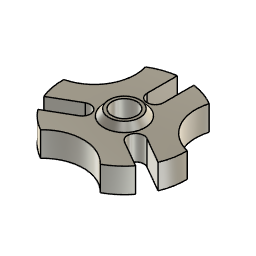
exercise13 (Autodesk Fusion 360 design; units mm, degrees)
Autodesk Fusion 360 part; units mm, degrees
sketch "草图1" plane through (0, 0, 0) normal (0, 0, 1) x (1, 0, 0)
  line L0 (0, 100) -> (0, -123.0461) construction
  line L1 (-180, 0) -> (103.1908, 0) construction
  arc A0 (14.5237, -26.25) -> (-14.5237, -26.25) centre (0, -40) ccw
  line L2 (-4, 29.7321) -> (-4, 15)
  line L3 (4, 15) -> (4, 29.7321)
  arc A1 (-4, 15) -> (0, 11) centre (0, 15) ccw
  arc A2 (0, 11) -> (4, 15) centre (0, 15) ccw
  line L4 (-14.9904, -4.0359) -> (-27.7488, -11.402)
  line L5 (-23.7488, -18.3302) -> (-10.9904, -10.9641)
  arc A3 (-10.9904, -10.9641) -> (-9.5263, -5.5) centre (-12.9904, -7.5) ccw
  arc A4 (-9.5263, -5.5) -> (-14.9904, -4.0359) centre (-12.9904, -7.5) ccw
  arc A5 (15.4713, 25.7029) -> (29.995, 0.5471) centre (34.641, 20) ccw
  line L6 (10.9904, -10.9641) -> (23.7488, -18.3302)
  line L7 (27.7488, -11.402) -> (14.9904, -4.0359)
  arc A6 (14.9904, -4.0359) -> (9.5263, -5.5) centre (12.9904, -7.5) ccw
  arc A7 (9.5263, -5.5) -> (10.9904, -10.9641) centre (12.9904, -7.5) ccw
  arc A8 (-29.995, 0.5471) -> (-15.4713, 25.7029) centre (-34.641, 20) ccw
  arc A9 (15.4713, 25.7029) -> (4, 29.7321) centre (0, 0) ccw
  arc A10 (-4, 29.7321) -> (-15.4713, 25.7029) centre (0, 0) ccw
  arc A11 (27.7488, -11.402) -> (29.995, 0.5471) centre (0, 0) ccw
  arc A12 (14.5237, -26.25) -> (23.7488, -18.3302) centre (0, 0) ccw
  arc A13 (-29.995, 0.5471) -> (-27.7488, -11.402) centre (0, 0) ccw
  arc A14 (-23.7488, -18.3302) -> (-14.5237, -26.25) centre (0, 0) ccw
  circle A15 centre (0, 0) radius 7.5
  circle A16 centre (0, 0) radius 10
  point P0 (-4, 11)
  point P1 (4, 11)
  dimension "d2" = 20
  dimension "d3" = 40
  dimension "d4" = 60
  dimension "d6" = 8
  dimension "d8" = 4
  dimension "d10" = 360
  dimension "d11" = 15
  dimension "d12" = 20
  constraint coincident A9.centre A10.centre
  constraint vertical L0
  constraint horizontal L1
  constraint coincident A0.start A13
  constraint symmetric L0 A0.end A0.start
  constraint coincident L2.start A13
  constraint coincident L3.end A13
  constraint symmetric L0 L2 L3
  constraint parallel L0 L3
  constraint coincident P0 L2
  constraint tangent L2 A1
  constraint coincident P1 L3
  constraint tangent L3 A2
  constraint equal A1 A2
  constraint coincident A1.end A2.start
  constraint concentric A9 A13
  constraint concentric A9 A10
  constraint concentric A11 A13
  constraint concentric A12 A13
  constraint concentric A13 A14
  constraint concentric A10 A15
  constraint concentric A11 A16
  measures "d2" radius of A0
  measures "d3" distance of A9.centre A0.centre
  measures "d4" diameter of A13
  measures "d6" distance of P0 P1
  measures "d8" radius of A1
  measures "d11" diameter of A15
  measures "d12" diameter of A16
extrude "拉伸1" add sketch "草图1" along normal blind 6 contours A0 L2 L3 A1 A2 L4 L5 A3 A4 A5 L6 L7 A6 A7 A8 A9 A10 A11 A12 A13 A14
sketch "草图2" plane through (0, 0, 0) normal (0, 0, 1) x (1, 0, 0)
  circle A0 centre (0, 0) radius 10
  constraint coincident A0.centre origin
ref_plane "工作平面1" through (0, 0, 9) normal (0, 0, 1) x (1, 0, 0)
sketch "草图3" plane through (0, 0, 9) normal (0, 0, 1) x (1, 0, 0)
  circle A0 centre (0, 0) radius 7.5
  circle A1 centre (0, 0) radius 6
  dimension "d16" = 15
  dimension "d17" = 12
  constraint coincident A0.centre A1.centre
  measures "d16" diameter of A0
  measures "d17" diameter of A1
extrude "拉伸2" add sketch "草图2" along normal blind 6
sketch "草图4" plane through (0, 0, 6) normal (0, 0, 1) x (-1, 0, 0)
  line L0 (10.9904, 10.9641) -> (23.7488, 18.3302)
  arc A0 (23.7488, 18.3302) -> (14.5237, 26.25) centre (0, 0) ccw
  arc A1 (-14.5237, 26.25) -> (14.5237, 26.25) centre (0, 40) ccw
  arc A2 (-14.5237, 26.25) -> (-23.7488, 18.3302) centre (0, 0) ccw
  line L1 (-23.7488, 18.3302) -> (-10.9904, 10.9641)
  arc A3 (-14.9904, 4.0359) -> (-10.9904, 10.9641) centre (-12.9904, 7.5) ccw
  line L2 (-14.9904, 4.0359) -> (-27.7488, 11.402)
  arc A4 (-27.7488, 11.402) -> (-29.995, -0.5471) centre (0, 0) ccw
  arc A5 (-15.4713, -25.7029) -> (-29.995, -0.5471) centre (-34.641, -20) ccw
  arc A6 (-15.4713, -25.7029) -> (-4, -29.7321) centre (0, 0) ccw
  line L3 (-4, -29.7321) -> (-4, -15)
  arc A7 (4, -15) -> (-4, -15) centre (0, -15) ccw
  line L4 (4, -15) -> (4, -29.7321)
  arc A8 (4, -29.7321) -> (15.4713, -25.7029) centre (0, 0) ccw
  arc A9 (29.995, -0.5471) -> (15.4713, -25.7029) centre (34.641, -20) ccw
  arc A10 (29.995, -0.5471) -> (27.7488, 11.402) centre (0, 0) ccw
  line L5 (27.7488, 11.402) -> (14.9904, 4.0359)
  arc A11 (10.9904, 10.9641) -> (14.9904, 4.0359) centre (12.9904, 7.5) ccw
  circle A12 centre (0, 0) radius 10
  constraint concentric A0 A12
loft "放样1" add profiles "草图4", "草图3" section 1 contours A12 section 2
extrude "拉伸3" cut sketch "草图3" against normal blind 21 contours A1
mirror "镜像1" about plane through (0, 0, 0) normal (0, 0, 1) of bodies 1 merged
